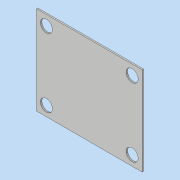
# Autodesk Inventor part: 自制垫片
Saved by Autodesk Inventor 2019 (Build 230136000, 136)
## iProperties
Created: 2020-12-08
Part Number: 自制垫片
Material: Generic
Document SubType Name: Modeling
Designer: Wang Hua
Density: 1 g/cm^3
Appearance: Default
Author: Wang Hua
Autodesk Inventor part; units mm, degrees
ref_plane "YZ Plane" through (0, 0, 0) normal (1, 0, 0) x (0, 1, 0)
ref_plane "XZ Plane" through (0, 0, 0) normal (0, 1, 0) x (-1, 0, 0)
ref_plane "XY Plane" through (0, 0, 0) normal (0, 0, 1) x (1, 0, 0)
sketch "草图1" plane through (0, 0, 0) normal (0, 0, 1) x (1, 0, 0)
  line L0 (18.5, -15.5) -> (-18.5, -15.5)
  line L1 (-18.5, -15.5) -> (-18.5, 15.5)
  line L2 (-18.5, 15.5) -> (18.5, 15.5)
  line L3 (18.5, 15.5) -> (18.5, -15.5)
  line L4 (18.5, -15.5) -> (-18.5, 15.5) construction
  line L5 (-18.5, -15.5) -> (18.5, 15.5) construction
  line L6 (0, 0) -> (-24.9379, 0) construction
  line L7 (0, 0) -> (0, 16.8364) construction
  point P0 (-15, 12)
  point P1 (-15, -12)
  point P2 (15, 12)
  point P3 (15, -12)
  dimension "d0" = 31
  dimension "d1" = 37
  dimension "d2" = 12
  dimension "d3" = 15
  constraints: 16 end point, 3 symmetric about line, 2 horizontal, 2 midpoint, 2 parallel, 1 perpendicular, 1 vertical
  measures "d0" distance of L0.end L1.end
  measures "d1" distance of L1.end L2.end
  measures "d2" vertical distance of L6.start point (-15, 12)
  measures "d3" horizontal distance of L6.start point (-15, 12)
extrude "拉伸1" add sketch "草图1" along normal blind 0.5
hole "孔1" at (-15, 12, 0) at (-15, -12, 0) at (15, 12, 0) at (15, -12, 0) direction (0, 0, 1) diameter 4.2 end through all
